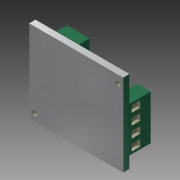
# Autodesk Inventor part: motorcontrol
Saved by Autodesk Inventor 2015 (Build 190159000, 159)
## iProperties
Created: 2015-01-29
Part Number: motorcontrol
Material: Generic
Document SubType Name: Modeling
Designer: 16111525
Density: 1 g/cm^3
Appearance: Low Pile - Gold
Author: 16111525
Autodesk Inventor part; units mm, degrees
ref_plane "YZ Plane" through (0, 0, 0) normal (1, 0, 0) x (0, 1, 0)
ref_plane "XZ Plane" through (0, 0, 0) normal (0, 1, 0) x (-1, 0, 0)
sketch "Sketch1" plane through (0, 0, 0) normal (0, 1, 0) x (-1, 0, 0)
  line L0 (5.8992, 33.2263) -> (-39.1008, 33.2263)
  line L1 (-39.1008, 33.2263) -> (-39.1008, -6.1737)
  line L2 (-39.1008, -6.1737) -> (5.8992, -6.1737)
  line L3 (5.8992, -6.1737) -> (5.8992, 33.2263)
  point P0 (0, 0)
  dimension "d0" = 45
  dimension "d1" = 39.4
  constraints: 8 end point, 2 parallel, 1 horizontal, 1 perpendicular
  measures "d0" distance of L2.end L1.end
  measures "d1" distance between parallel lines of L2 L0
extrude "Extrusion1" add sketch "Sketch1" along normal blind 3
sketch "Sketch2" plane through (0, 3, 0) normal (0, 1, 0) x (1, 0, 0)
  line L0 (-5.8992, 6.1737) -> (-5.8992, -33.2263) projected
  line L1 (-5.8992, -8.1763) -> (0.5008, -8.1763)
  line L2 (0.5008, -8.1763) -> (0.5008, -18.8763)
  line L3 (0.5008, -18.8763) -> (-5.8992, -18.8763)
  line L4 (-5.8992, -18.8763) -> (-5.8992, -8.1763)
  line L5 (39.1008, 6.1737) -> (-5.8992, 6.1737) projected
  line L6 (-5.8992, -33.2263) -> (39.1008, -33.2263) projected
  point P0 (0, 0)
  dimension "d4" = 14.35
  dimension "d5" = 14.35
  dimension "d6" = 6.4
  constraints: 8 end point, 2 parallel, 1 horizontal, 1 perpendicular, 1 point on line
  measures "d4" distance between parallel lines of L5 L1
  measures "d5" distance between parallel lines of L6 L3
  measures "d6" distance between parallel lines of L2 L0
extrude "Extrusion2" add sketch "Sketch2" along normal blind 10.2
sketch "Sketch3" plane through (0, 13.2, 0) normal (0, 1, 0) x (1, 0, 0)
  circle A0 centre (-2.6992, -16.3763) radius 1.85
  line L0 (-5.8992, -18.8763) -> (0.5008, -18.8763) projected
  circle A1 centre (-2.6992, -10.6763) radius 1.85
  line L1 (0.5008, -8.1763) -> (-5.8992, -8.1763) projected
  line L2 (0.5008, -18.8763) -> (0.5008, -8.1763) projected
  line L3 (-5.8992, -8.1763) -> (-5.8992, -18.8763) projected
  point P0 (0, 0)
  dimension "d10" = 3.7
  dimension "d12" = 2.5
  dimension "d13" = 3.7
  dimension "d14" = 2.5
  dimension "d17" = 3.2
  dimension "d18" = 3.2
  constraints: 2 centre point
  measures "d10" diameter of A0
  measures "d12" distance from line of L0 A0.centre
  measures "d13" diameter of A1
  measures "d14" distance from line of L1 A1.centre
  measures "d17" distance from line of L3 A0.centre
  measures "d18" distance from line of L3 A1.centre
extrude "Extrusion3" cut sketch "Sketch3" against normal blind 1.4 contours A0 | A1
sketch "Sketch4" plane through (0, 3, 0) normal (0, 1, 0) x (1, 0, 0)
  line L0 (-0.8992, -21.8263) -> (9.8008, -21.8263)
  line L1 (9.8008, -21.8263) -> (9.8008, -28.2263)
  line L2 (9.8008, -28.2263) -> (-0.8992, -28.2263)
  line L3 (-0.8992, -28.2263) -> (-0.8992, -21.8263)
  line L4 (-5.8992, -33.2263) -> (39.1008, -33.2263) projected
  line L5 (-5.8992, -18.8763) -> (-5.8992, -33.2263) projected
  line L6 (-0.8992, 1.1737) -> (9.8008, 1.1737)
  line L7 (9.8008, 1.1737) -> (9.8008, -5.2263)
  line L8 (9.8008, -5.2263) -> (-0.8992, -5.2263)
  line L9 (-0.8992, -5.2263) -> (-0.8992, 1.1737)
  line L10 (-5.8992, 6.1737) -> (-5.8992, -8.1763) projected
  line L11 (39.1008, 6.1737) -> (-5.8992, 6.1737) projected
  circle A0 centre (1.6008, -25.0263) radius 1.85
  circle A1 centre (7.3008, -25.0263) radius 1.85
  circle A2 centre (1.6008, -2.0263) radius 1.85
  circle A3 centre (7.3008, -2.0263) radius 1.85
  point P0 (0, 0)
  dimension "d21" = 5
  dimension "d22" = 5
  dimension "d23" = 6.4
  dimension "d24" = 10.7
  dimension "d25" = 10.7
  dimension "d26" = 5
  dimension "d27" = 5
  dimension "d28" = 6.4
  dimension "d29" = 3.7
  dimension "d30" = 2.5
  dimension "d31" = 3.2
  dimension "d32" = 3.7
  dimension "d33" = 2.5
  dimension "d34" = 3.2
  dimension "d35" = 3.7
  dimension "d36" = 3.7
  dimension "d37" = 2.5
  dimension "d38" = 3.2
  dimension "d39" = 3.2
  dimension "d40" = 2.5
  constraints: 16 end point, 4 centre point, 4 parallel, 2 horizontal, 2 perpendicular
  measures "d21" distance between parallel lines of L4 L2
  measures "d22" distance between parallel lines of L5 L3
  measures "d23" distance between parallel lines of L0 L2
  measures "d24" distance between parallel lines of L1 L3
  measures "d25" distance between parallel lines of L7 L9
  measures "d26" distance between parallel lines of L10 L9
  measures "d27" distance between parallel lines of L6 L11
  measures "d28" distance between parallel lines of L8 L6
  measures "d29" diameter of A0
  measures "d30" distance from line of A0.centre L3
  measures "d31" distance from line of L2 A0.centre
  measures "d32" diameter of A1
  measures "d33" distance from line of L1 A1.centre
  measures "d34" distance from line of L2 A1.centre
  measures "d35" diameter of A2
  measures "d36" diameter of A3
  measures "d37" distance from line of L9 A2.centre
  measures "d38" distance from line of L8 A2.centre
  measures "d39" distance from line of L8 A3.centre
  measures "d40" distance from line of A3.centre L7
extrude "Extrusion4" add sketch "Sketch4" along normal blind 10.2 contours L0 L1 L2 L3 | L6 L7 L8 L9 | A0 | A1 | A2 | A3
sketch "Sketch5" plane through (0, 13.2, 0) normal (0, 1, 0) x (1, 0, 0)
  circle A0 centre (1.6008, -2.0263) radius 1.85
  circle A1 centre (7.3008, -2.0263) radius 1.85
  line L0 (-0.8992, 1.1737) -> (-0.8992, -5.2263) projected
  line L1 (-0.8992, -5.2263) -> (9.8008, -5.2263) projected
  line L2 (9.8008, -5.2263) -> (9.8008, 1.1737) projected
  point P0 (0, 0)
  dimension "d43" = 3.7
  dimension "d44" = 3.7
  dimension "d45" = 2.5
  dimension "d46" = 3.2
  dimension "d47" = 3.2
  dimension "d48" = 2.5
  constraints: 2 centre point
  measures "d43" diameter of A0
  measures "d44" diameter of A1
  measures "d45" distance from line of L0 A0.centre
  measures "d46" distance from line of L1 A0.centre
  measures "d47" distance from line of L1 A1.centre
  measures "d48" distance from line of L2 A1.centre
extrude "Extrusion5" cut sketch "Sketch5" against normal blind 1.4
sketch "Sketch6" plane through (0, 13.2, 0) normal (0, 1, 0) x (1, 0, 0)
  circle A0 centre (1.6008, -25.0263) radius 1.85
  circle A1 centre (7.3008, -25.0263) radius 1.85
  line L0 (9.8008, -21.8263) -> (-0.8992, -21.8263) projected
  line L1 (-0.8992, -21.8263) -> (-0.8992, -28.2263) projected
  line L2 (9.8008, -28.2263) -> (9.8008, -21.8263) projected
  point P0 (0, 0)
  dimension "d51" = 3.7
  dimension "d52" = 3.7
  dimension "d53" = 3.2
  dimension "d54" = 2.5
  dimension "d55" = 3.2
  dimension "d56" = 2.5
  constraints: 2 centre point
  measures "d51" diameter of A0
  measures "d52" diameter of A1
  measures "d53" distance from line of L0 A0.centre
  measures "d54" distance from line of L1 A0.centre
  measures "d55" distance from line of L0 A1.centre
  measures "d56" distance from line of L2 A1.centre
extrude "Extrusion6" cut sketch "Sketch6" against normal blind 1.4
sketch "Sketch7" plane through (0, 3, 0) normal (0, 1, 0) x (1, 0, 0)
  line L0 (39.1008, -33.2263) -> (39.1008, 6.1737) projected
  line L1 (39.1008, -20.8263) -> (32.7008, -20.8263)
  line L2 (32.7008, -20.8263) -> (32.7008, 0.5737)
  line L3 (32.7008, 0.5737) -> (39.1008, 0.5737)
  line L4 (39.1008, 0.5737) -> (39.1008, -20.8263)
  line L5 (39.1008, 6.1737) -> (-5.8992, 6.1737) projected
  point P0 (0, 0)
  dimension "d59" = 6.4
  dimension "d60" = 21.4
  dimension "d61" = 5.6
  constraints: 8 end point, 2 parallel, 1 horizontal, 1 perpendicular, 1 point on line
  measures "d59" distance of L2.end L3.end
  measures "d60" distance between parallel lines of L3 L1
  measures "d61" distance between parallel lines of L5 L3
extrude "Extrusion7" add sketch "Sketch7" along normal blind 10.2
sketch "Sketch8" plane through (0, 13.2, 0) normal (0, 1, 0) x (1, 0, 0)
  circle A0 centre (35.9008, -1.9263) radius 1.85
  circle A1 centre (35.9008, -7.6263) radius 1.85
  circle A2 centre (35.9008, -12.6263) radius 1.85
  circle A3 centre (35.9008, -18.3263) radius 1.85
  line L0 (39.1008, -20.8263) -> (39.1008, 0.5737) projected
  line L1 (39.1008, 0.5737) -> (32.7008, 0.5737) projected
  line L2 (32.7008, -20.8263) -> (39.1008, -20.8263) projected
  point P0 (0, 0)
  dimension "d39" = 3.2
  dimension "d64" = 3.7
  dimension "d65" = 3.7
  dimension "d66" = 3.7
  dimension "d67" = 3.7
  dimension "d68" = 3.2
  dimension "d69" = 2.5
  dimension "d70" = 3.2
  dimension "d71" = 2.5
  dimension "d72" = 5.7
  dimension "d73" = 3.2
  dimension "d74" = 5.7
  dimension "d75" = 3.2
  constraints: 4 centre point
  measures "d64" diameter of A0
  measures "d65" diameter of A1
  measures "d66" diameter of A2
  measures "d67" diameter of A3
  measures "d68" distance from line of L0 A0.centre
  measures "d69" distance from line of L1 A0.centre
  measures "d70" distance from line of L0 A3.centre
  measures "d71" distance from line of L2 A3.centre
  measures "d72" distance of A1.centre A0.centre
  measures "d73" distance from line of L0 A1.centre
  measures "d74" distance of A2.centre A3.centre
  measures "d75" distance from line of L0 A2.centre
extrude "Extrusion8" cut sketch "Sketch8" against normal blind 1.4
sketch "Sketch10" plane through (9.8008, 3, -1.1737) normal (0, 0, -1) x (-1, 0, 0)
  line L0 (1.1, 5.2) -> (4.25, 5.2)
  line L1 (4.25, 5.2) -> (4.25, 1.1)
  line L2 (4.25, 1.1) -> (1.1, 1.1)
  line L3 (1.1, 1.1) -> (1.1, 5.2)
  line L4 (0, 0) -> (0, 10.2) projected
  line L5 (10.7, 0) -> (0, 0) projected
  line L6 (6.45, 5.2) -> (9.6, 5.2)
  line L7 (9.6, 5.2) -> (9.6, 1.1)
  line L8 (9.6, 1.1) -> (6.45, 1.1)
  line L9 (6.45, 1.1) -> (6.45, 5.2)
  line L10 (10.7, 0) -> (10.7, 10.2) projected
  point P0 (9.8008, -3)
  dimension "d78" = 1.1
  dimension "d79" = 1.1
  dimension "d80" = 4.1
  dimension "d81" = 1.1
  dimension "d82" = 2.2
  dimension "d83" = 4.1
  dimension "d84" = 1.1
  dimension "d85" = 3.15
  constraints: 16 end point, 4 parallel, 2 horizontal, 2 perpendicular
  measures "d78" distance between parallel lines of L4 L3
  measures "d79" distance between parallel lines of L5 L2
  measures "d80" distance between parallel lines of L0 L2
  measures "d81" distance between parallel lines of L5 L8
  measures "d82" distance between parallel lines of L1 L9
  measures "d83" distance between parallel lines of L8 L6
  measures "d84" distance between parallel lines of L10 L7
  measures "d85" distance between parallel lines of L1 L3
extrude "Extrusion9" cut sketch "Sketch10" against normal blind 1.4
sketch "Sketch11" plane through (-5.8992, 0, -6.1737) normal (-1, 0, 0) x (0, 0, 1)
  line L0 (15.45, 8.2) -> (18.6, 8.2)
  line L1 (18.6, 8.2) -> (18.6, 4.1)
  line L2 (18.6, 4.1) -> (15.45, 4.1)
  line L3 (15.45, 4.1) -> (15.45, 8.2)
  line L4 (20.8, 8.2) -> (23.95, 8.2)
  line L5 (23.95, 8.2) -> (23.95, 4.1)
  line L6 (23.95, 4.1) -> (20.8, 4.1)
  line L7 (20.8, 4.1) -> (20.8, 8.2)
  line L8 (14.35, 3) -> (14.35, 13.2) projected
  line L9 (25.05, 3) -> (25.05, 13.2) projected
  line L10 (14.35, 3) -> (25.05, 3)
  line L11 (0, 3) -> (14.35, 3) projected
  point P0 (6.1737, 0)
  dimension "d88" = 1.1
  dimension "d89" = 2.2
  dimension "d90" = 1.1
  dimension "d91" = 1.1
  dimension "d92" = 3.15
  dimension "d93" = 4.1
  constraints: 18 end point, 4 parallel, 2 horizontal, 2 perpendicular, 2 point on line, 1 collinear
  measures "d88" distance between parallel lines of L8 L3
  measures "d89" distance between parallel lines of L7 L1
  measures "d90" distance between parallel lines of L9 L5
  measures "d91" distance between parallel lines of L10 L2
  measures "d92" distance between parallel lines of L1 L3
  measures "d93" distance between parallel lines of L2 L0
extrude "Extrusion10" cut sketch "Sketch11" against normal blind 1.4
sketch "Sketch12" plane through (-0.8992, 3, 28.2263) normal (0, 0, 1) x (1, 0, 0)
  line L0 (1.1, 5.2) -> (4.25, 5.2)
  line L1 (4.25, 5.2) -> (4.25, 1.1)
  line L2 (4.25, 1.1) -> (1.1, 1.1)
  line L3 (1.1, 1.1) -> (1.1, 5.2)
  line L4 (6.45, 5.2) -> (9.6, 5.2)
  line L5 (9.6, 5.2) -> (9.6, 1.1)
  line L6 (9.6, 1.1) -> (6.45, 1.1)
  line L7 (6.45, 1.1) -> (6.45, 5.2)
  line L8 (10.7, 0) -> (10.7, 10.2) projected
  line L9 (-5, 0) -> (40, 0) projected
  point P0 (0.8992, -3)
  dimension "d96" = 3.15
  dimension "d97" = 3.15
  dimension "d98" = 2.2
  dimension "d99" = 1.1
  dimension "d100" = 4.1
  dimension "d101" = 1.1
  constraints: 16 end point, 4 parallel, 2 horizontal, 2 perpendicular, 2 point on line
  measures "d96" distance of L1.end L2.end
  measures "d97" distance of L5.end L6.end
  measures "d98" distance between parallel lines of L7 L1
  measures "d99" distance between parallel lines of L8 L5
  measures "d100" distance between parallel lines of L6 L4
  measures "d101" distance between parallel lines of L9 L2
extrude "Extrusion11" cut sketch "Sketch12" against normal blind 1.4
sketch "Sketch13" plane through (39.1008, 0, 33.2263) normal (1, 0, 0) x (0, 0, -1)
  line L0 (15.45, 4.1) -> (18.6, 4.1) projected
  line L1 (13.5, 8.2) -> (16.65, 8.2)
  line L2 (16.65, 8.2) -> (16.65, 4.1)
  line L3 (16.65, 4.1) -> (13.5, 4.1)
  line L4 (13.5, 4.1) -> (13.5, 8.2)
  line L5 (18.85, 8.2) -> (22, 8.2)
  line L6 (22, 8.2) -> (22, 4.1)
  line L7 (22, 4.1) -> (18.85, 4.1)
  line L8 (18.85, 4.1) -> (18.85, 8.2)
  line L9 (12.4, 3) -> (12.4, 13.2) projected
  line L10 (12.4, 3) -> (34.1653, 3)
  line L11 (33.8, 3) -> (39.4, 3) projected
  line L12 (33.8, 3) -> (33.8, 13.2) projected
  line L13 (24.2, 8.2) -> (27.35, 8.2)
  line L14 (27.35, 8.2) -> (27.35, 4.1)
  line L15 (27.35, 4.1) -> (24.2, 4.1)
  line L16 (24.2, 4.1) -> (24.2, 8.2)
  line L17 (29.55, 8.2) -> (32.7, 8.2)
  line L18 (32.7, 8.2) -> (32.7, 4.1)
  line L19 (32.7, 4.1) -> (29.55, 4.1)
  line L20 (29.55, 4.1) -> (29.55, 8.2)
  point P0 (33.2263, 0)
  dimension "d104" = 3.15
  dimension "d105" = 3.15
  dimension "d108" = 1.1
  dimension "d111" = 2.2
  dimension "d112" = 4.1
  dimension "d113" = 4.1
  dimension "d121" = 3.15
  dimension "d122" = 3.15
  dimension "d123" = 1.1
  dimension "d124" = 2.2
  dimension "d125" = 1.1
  dimension "d126" = 1.1
  dimension "d127" = 4.1
  constraints: 34 end point, 8 parallel, 4 horizontal, 4 perpendicular, 4 point on line
  measures "d104" distance of L2.end L3.end
  measures "d105" distance of L6.end L7.end
  measures "d108" distance between parallel lines of L9 L4
  measures "d111" distance between parallel lines of L2 L8
  measures "d112" distance between parallel lines of L3 L1
  measures "d113" distance between parallel lines of L7 L5
  measures "d121" distance of L14.end L15.end
  measures "d122" distance of L18.end L19.end
  measures "d123" distance between parallel lines of L12 L18
  measures "d124" distance between parallel lines of L20 L14
  measures "d125" distance between parallel lines of L10 L19
  measures "d126" distance between parallel lines of L10 L15
  measures "d127" distance between parallel lines of L15 L13
extrude "Extrusion12" cut sketch "Sketch13" against normal blind 1.4
ref_plane "Work Plane1" through (2.5008, 3, 18.8763) normal (1, 0, 0) x (0, 0, -1)
sketch "Sketch17" plane through (2.5008, 3, 18.8763) normal (1, 0, 0) x (0, 0, -1)
  circle A0 centre (5.0355, 4.4753) radius 4.2987
  point P0 (18.8763, -3)
  constraints: 1 centre point
extrude "Extrusion13" add sketch "Sketch17" along normal blind 22
sketch "Sketch18" plane through (0, 3, 0) normal (0, 1, 0) x (1, 0, 0)
  line L0 (33.4369, -29.0517) -> (19.8703, -29.0517)
  line L1 (19.8703, -29.0517) -> (19.8703, -23.9814)
  line L2 (19.8703, -23.9814) -> (33.4369, -23.9814)
  line L3 (33.4369, -23.9814) -> (33.4369, -29.0517)
  point P0 (0, 0)
  constraints: 8 end point, 2 parallel, 1 horizontal, 1 perpendicular
extrude "Extrusion14" add sketch "Sketch18" along normal blind 2
sketch "Sketch19" plane through (0, 3, 0) normal (0, 1, 0) x (1, 0, 0)
  circle A0 centre (-3.2492, 2.8237) radius 1.15
  line L0 (39.1008, 6.1737) -> (-5.8992, 6.1737) projected
  line L1 (-5.8992, 6.1737) -> (-5.8992, -8.1763) projected
  circle A1 centre (36.6508, -29.4203) radius 1.15
  line L2 (-5.8992, -33.2263) -> (39.1008, -33.2263) projected
  line L3 (39.1008, -33.2263) -> (39.1008, -20.8263) projected
  point P0 (0, 0)
  dimension "d135" = 2.3
  dimension "d136" = 3.35
  dimension "d137" = 2.65
  dimension "d138" = 2.3
  dimension "d139" = 51.3
  dimension "d141" = 2.45
  constraints: 2 centre point
  measures "d135" diameter of A0
  measures "d136" distance from line of L0 A0.centre
  measures "d137" distance from line of L1 A0.centre
  measures "d138" diameter of A1
  measures "d139" distance of A1.centre A0.centre
  measures "d141" distance from line of L3 A1.centre
extrude "Extrusion15" cut sketch "Sketch19" against normal blind 3
body "Solid1"
